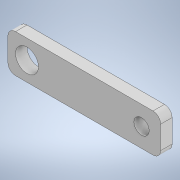
# Autodesk Inventor part: лапка сервы
Saved by Autodesk Inventor 2020.1 (Build 241239000, 239)
## iProperties
Created: 2022-04-06
Part Number: лапка сервы
Material: Типовые
Document SubType Name: Modeling
Designer: User
Density: 1 g/cm^3
Appearance: По умолчанию
Author: User
Autodesk Inventor part; units mm, degrees
ref_plane "YZ Plane" through (0, 0, 0) normal (1, 0, 0) x (0, 1, 0)
ref_plane "XZ Plane" through (0, 0, 0) normal (0, 1, 0) x (-1, 0, 0)
ref_plane "XY Plane" through (0, 0, 0) normal (0, 0, 1) x (1, 0, 0)
sketch "Эскиз1" plane through (0, 0, 0) normal (0, 0, 1) x (1, 0, 0)
  line L0 (-4.7967, -2.561) -> (35.2033, -2.561)
  line L1 (35.2033, -2.561) -> (35.2033, 7.439)
  line L2 (35.2033, 7.439) -> (-4.7967, 7.439)
  line L3 (-4.7967, 7.439) -> (-4.7967, -2.561)
  point P0 (0, 0)
  dimension "d0" = 10
  dimension "d1" = 40
  constraints: 8 end point, 2 parallel, 1 horizontal, 1 perpendicular
  measures "d0" distance of L2.end L0.start
  measures "d1" distance of L1.end L2.end
extrude "Выдавливание1" add sketch "Эскиз1" along normal blind 3
sketch "Эскиз2" plane through (0, 0, 3) normal (0, 0, 1) x (1, 0, 0)
  line L0 (-4.7967, 7.439) -> (-4.7967, -2.561) projected
  circle A0 centre (0.2033, 2.439) radius 3
  circle A1 centre (30.2033, 2.439) radius 2
  line L1 (35.2033, -2.561) -> (35.2033, 7.439) projected
  point P0 (0, 0)
  point P1 (-4.7967, 2.439)
  dimension "d4" = 6
  dimension "d5" = 5
  dimension "d6" = 4
  dimension "d7" = 5
  constraints: 2 centre point, 1 midpoint
  measures "d4" diameter of A0
  measures "d5" distance of A0.centre point (-4.797, 2.439)
  measures "d6" diameter of A1
  measures "d7" distance from line of L1 A1.centre
extrude "Выдавливание2" cut sketch "Эскиз2" against normal blind 10
fillet "Сопряжение1" radius 2 4 edges at (-4.7967, 7.439, 1.5) (-4.7967, -2.561, 1.5) (35.2033, -2.561, 1.5) (35.2033, 7.439, 1.5)
